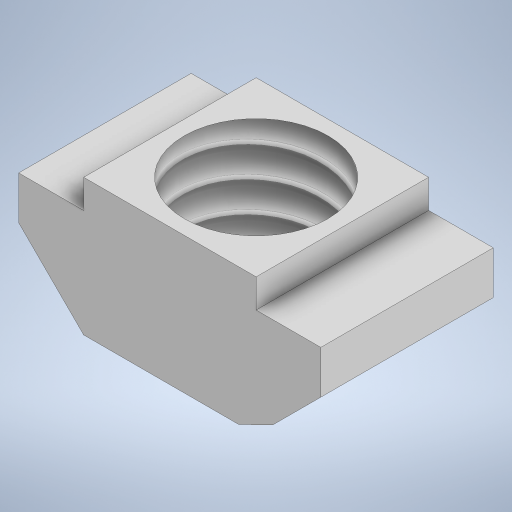
# Autodesk Inventor part: M5 Model
Saved by Autodesk Inventor 2023.5 (Build 275446000, 446)
## iProperties
Created: 2024-07-24
Part Number: M5 Model
Material: Generic
Document SubType Name: Modeling
Designer: punny
Density: 1 g/cm^3
Appearance: Default
Author: punny
Autodesk Inventor part; units mm, degrees
ref_plane "YZ Plane" through (0, 0, 0) normal (1, 0, 0) x (0, 1, 0)
ref_plane "XZ Plane" through (0, 0, 0) normal (0, 1, 0) x (-1, 0, 0)
ref_plane "XY Plane" through (0, 0, 0) normal (0, 0, 1) x (1, 0, 0)
sketch "Sketch1" plane through (0, 0, 0) normal (0, 0, 1) x (1, 0, 0)
  line L0 (0.6988, 10.196) -> (0.6988, 11.196)
  line L1 (0.6988, 11.196) -> (6.6988, 11.196)
  line L2 (6.6988, 11.196) -> (6.6988, 10.196)
  line L3 (6.6988, 10.196) -> (8.9488, 10.196)
  line L4 (8.9488, 10.196) -> (8.9488, 8.696)
  line L5 (8.9488, 8.696) -> (7.2785, 7.0257)
  line L6 (8.9488, 8.696) -> (11.311, 8.696) construction
  line L7 (7.2785, 7.0257) -> (6.0988, 6.446)
  line L8 (0.6988, 10.196) -> (-1.5618, 10.196)
  line L9 (-1.5618, 10.196) -> (-1.5618, 8.696)
  line L10 (-1.5618, 8.696) -> (0.6988, 6.446)
  line L11 (0.6988, 6.446) -> (6.0988, 6.446)
  point P0 (0, 0)
  point P1 (-6.8565, -7.9644)
  dimension "d0" = 1
  dimension "d1" = 6
  dimension "d2" = 2.25
  dimension "d3" = 1.5
  dimension "d4" = 2.3622
  dimension "d5" = 135
  dimension "d6" = 2.2606
  constraints: 24 end point, 4 vertical, 3 horizontal, 1 equal length, 1 perpendicular
  measures "d0" distance of L0.start L0.end
  measures "d1" distance of L0.end L1.end
  measures "d2" distance of L2.end L3.end
  measures "d3" distance of L3.end L4.end
  measures "d4" distance of L4.end L5.end
  measures "d5" angle of L5 L6
  measures "d6" distance of L0.start L8.end
extrude "Extrusion1" add sketch "Sketch1" along normal blind 6
sketch "Sketch5" plane through (0.6988, 11.196, 0) normal (0, 1, 0) x (1, 0, 0)
  line L0 (-2.2606, 0) -> (0, 0) projected
  line L1 (6, 0) -> (6, -6) projected
  line L2 (0, 0) -> (6, 0)
  line L3 (6, 0) -> (6, -6)
  line L4 (6, -6) -> (0, -6)
  line L5 (0, -6) -> (0, 0)
  circle A0 centre (3, -3) radius 2.5
  point P0 (-0.6988, 0)
  dimension "d19" = 5
  constraints: 8 end point, 2 parallel, 1 centre point, 1 horizontal, 1 perpendicular
  measures "d19" diameter of A0
hole "Hole2" at (3.6988, 11.196, 3) direction (0, -1, 0) diameter 5 end through all
thread "Thread2" size "12-24 UNC" class "2B" standard "ANSI Unified Screw Threads" full length
body "Solid1"
